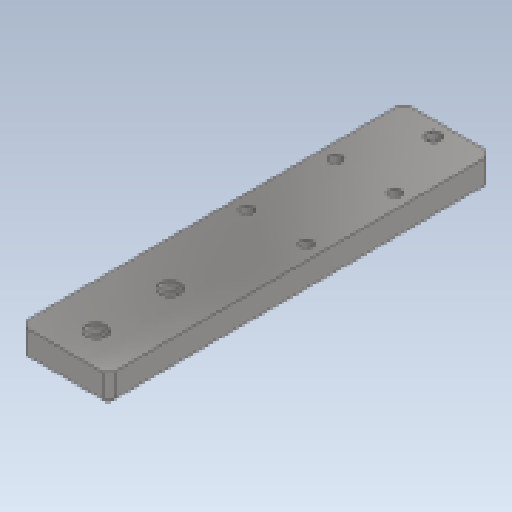
# Autodesk Inventor part: Horizontal_support
Saved by Autodesk Inventor 2025.2 (Build 292293000, 293)
## iProperties
Created: 2025-05-01
Part Number: Horizontal_support
Material: Stainless Steel
Document SubType Name: Modeling
Designer: Sergio Quintero
Density: 8 g/cm^3
Appearance: Semi-Polished
Author: Sergio Quintero
Autodesk Inventor part; units mm, degrees
ref_plane "YZ Plane" through (0, 0, 0) normal (1, 0, 0) x (0, 1, 0)
ref_plane "XZ Plane" through (0, 0, 0) normal (0, 1, 0) x (-1, 0, 0)
ref_plane "XY Plane" through (0, 0, 0) normal (0, 0, 1) x (1, 0, 0)
sketch "Sketch1" plane through (0, 0, 0) normal (0, 1, 0) x (-1, 0, 0)
  line L0 (-15, -65) -> (15, -65)
  line L1 (15, -65) -> (15, 65)
  line L2 (15, 65) -> (-15, 65)
  line L3 (-15, 65) -> (-15, -65)
  line L4 (-15, -65) -> (15, 65) construction
  line L5 (15, -65) -> (-15, 65) construction
  point P0 (0, 0)
  dimension "d0" = 30
  dimension "d1" = 130
  constraints: 12 end point, 2 midpoint, 2 parallel, 1 horizontal, 1 perpendicular
  measures "d0" distance of L2.end L1.end
  measures "d1" distance of L1.end L0.end
extrude "Extrusion1" add sketch "Sketch1" along normal blind 10
sketch "Sketch2" plane through (0, 10, 0) normal (0, 1, 0) x (1, 0, 0)
  line L0 (15, 65) -> (-15, 65) projected
  point P0 (0, 0)
  point P1 (0, -29)
  point P2 (0, -54)
  dimension "d4" = 94
  dimension "d5" = 25
  measures "d4" distance from line of L0 point (0, -29)
  measures "d5" distance of point (0, -54) point (0, -29)
hole "Hole1" at (0, 10, 29) at (0, 10, 54) direction (0, -1, 0) diameter 6.647 depth 22.2 tip angle 118 thread size "M8x1.25" class "6H" standard "ISO Metric profile"
sketch "Sketch3" plane through (0, 0, 0) normal (0, -1, 0) x (1, 0, 0)
  line L0 (15, -65) -> (-15, -65) projected
  line L1 (-15, -65) -> (-15, 65) projected
  point P0 (0, 0)
  point P1 (0, -60)
  dimension "d13" = 5
  dimension "d14" = 15
  measures "d13" distance from line of point (0, -60) L0
  measures "d14" distance from line of L1 point (0, -60)
hole "Hole2" at (0, 0, -60) direction (0, 1, 0) diameter 4.917 end through all thread size "M6x1" class "6H" standard "ISO Metric profile"
sketch "Sketch4" plane through (0, 0, 0) normal (0, -1, 0) x (1, 0, 0)
  line L0 (10, -37) -> (-10, -37) construction
  line L1 (-10, -37) -> (-10, -7) construction
  line L2 (-10, -7) -> (10, -7) construction
  line L3 (10, -7) -> (10, -37) construction
  line L4 (15, -65) -> (-15, -65) construction
  line L5 (15, 65) -> (15, -65) construction
  point P0 (0, 0)
  dimension "d22" = 20
  dimension "d23" = 30
  dimension "d24" = 28
  dimension "d25" = 5
  constraints: 8 end point, 4 coincident, 2 parallel, 1 horizontal, 1 perpendicular
  measures "d22" distance of L1.end L2.end
  measures "d23" distance of L0.end L1.end
  measures "d24" distance between parallel lines of L4 L0
  measures "d25" distance between parallel lines of L5 L3
hole "Hole3" at (10, 0, -37) at (-10, 0, -37) at (-10, 0, -7) at (10, 0, -7) direction (0, 1, 0) diameter 4.134 end through all thread size "M5x0.8" class "6H" standard "ISO Metric profile"
chamfer "Chamfer1" distance 2 angle 45 8 edges at (15, 5, -65) (-15, 5, -65) (15, 5, 65) (15, 0, 0) (0, 0, -65) (-15, 0, 0) (0, 0, 65) (-15, 5, 65)
body "Solid1"
